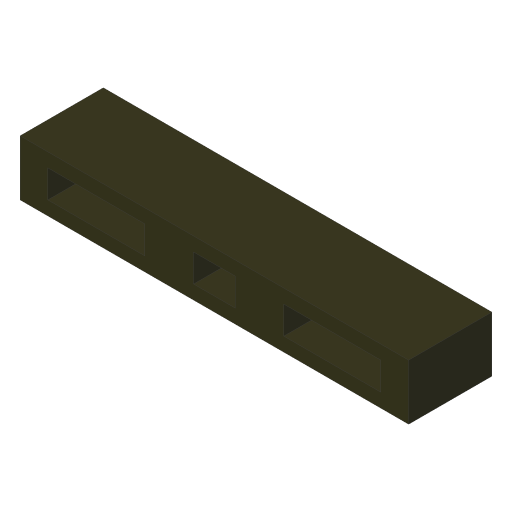
# Autodesk Inventor part: Fixture
Saved by Autodesk Inventor 2023.4 (Build 274418000, 418)
## iProperties
Created: 2024-02-27
Part Number: Fixture
Material: Generic
Document SubType Name: Modeling
Designer: josep
Density: 1 g/cm^3
Appearance: Default
Author: josep
Autodesk Inventor part; units mm, degrees
ref_plane "YZ Plane" through (0, 0, 0) normal (1, 0, 0) x (0, 1, 0)
ref_plane "XZ Plane" through (0, 0, 0) normal (0, 1, 0) x (-1, 0, 0)
ref_plane "XY Plane" through (0, 0, 0) normal (0, 0, 1) x (1, 0, 0)
sketch "Sketch1" plane through (0, 0, 0) normal (0, 0, 1) x (1, 0, 0)
  line L0 (-35, 5) -> (35, 5)
  line L1 (35, 5) -> (35, -5)
  line L2 (35, -5) -> (-35, -5)
  line L3 (-35, -5) -> (-35, 5)
  line L4 (-30, 2.5) -> (-12.5, 2.5)
  line L5 (-12.5, 2.5) -> (-12.5, -2.5)
  line L6 (-12.5, -2.5) -> (-30, -2.5)
  line L7 (-30, -2.5) -> (-30, 2.5)
  line L8 (12.5, 2.5) -> (30, 2.5)
  line L9 (30, 2.5) -> (30, -2.5)
  line L10 (30, -2.5) -> (12.5, -2.5)
  line L11 (12.5, -2.5) -> (12.5, 2.5)
  line L12 (-3.75, 2.5) -> (3.75, 2.5)
  line L13 (3.75, 2.5) -> (3.75, -2.5)
  line L14 (3.75, -2.5) -> (-3.75, -2.5)
  line L15 (-3.75, -2.5) -> (-3.75, 2.5)
  point P0 (0, 0)
  dimension "d0" = 70
  dimension "d1" = 5
  dimension "d2" = 10
  dimension "d3" = 35
  dimension "d5" = 5
  dimension "d6" = 5
  dimension "d7" = 5
  dimension "d8" = 17.5
  dimension "d9" = 17.5
  dimension "d10" = 2.5
  dimension "d13" = 7.5
  dimension "d14" = 5
  dimension "d15" = 3.75
  dimension "d16" = 2.5
  constraints: 32 end point, 8 parallel, 4 horizontal, 4 perpendicular, 2 point on line
  measures "d0" distance of L1.end L2.end
  measures "d1" vertical distance of L2.end point (0, 0)
  measures "d2" distance of L2.end L0.start
  measures "d3" horizontal distance of L0.start point (0, 0)
  measures "d5" horizontal distance of L2.end L6.end
  measures "d6" horizontal distance of L0.end L8.end
  measures "d7" distance of L6.end L4.start
  measures "d8" distance of L4.start L4.end
  measures "d9" distance of L8.start L8.end
  measures "d10" distance between parallel lines of L2 L10
  measures "d13" distance of L12.start L12.end
  measures "d14" distance of L12.end L13.end
  measures "d15" horizontal distance of L12.start point (0, 0)
  measures "d16" vertical distance of L12.start point (0, 0)
extrude "Extrusion1" add sketch "Sketch1" along normal blind 15
body "Solid1"
